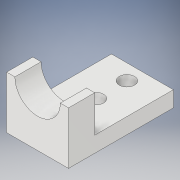
# Autodesk Inventor part: IndicatorLightMount
Saved by Autodesk Inventor 2018 (Build 220112000, 112)
## iProperties
Created: 2019-04-15
Part Number: IndicatorLightMount
Material: Generic
Document SubType Name: Modeling
Designer: anirudh
Density: 1 g/cm^3
Appearance: White
Mass: 2.43229 g
Surface Area: 18.7803 cm^2
Volume: 2.43229 cm^3
Author: anirudh
Autodesk Inventor part; units mm, degrees
ref_plane "YZ Plane" through (0, 0, 0) normal (1, 0, 0) x (0, 1, 0)
ref_plane "XZ Plane" through (0, 0, 0) normal (0, 1, 0) x (-1, 0, 0)
ref_plane "XY Plane" through (0, 0, 0) normal (0, 0, 1) x (1, 0, 0)
sketch "Sketch1" plane through (0, 0, 0) normal (0, 1, 0) x (-1, 0, 0)
  line L0 (0, 0) -> (15, 0)
  line L1 (15, 0) -> (15, 25.4)
  line L2 (15, 25.4) -> (0, 25.4)
  line L3 (0, 25.4) -> (0, 0)
  dimension "d0" = 15
  dimension "d1" = 25.4
  constraints: 8 end point, 2 parallel, 1 horizontal, 1 perpendicular
  measures "d0" distance of L2.end L1.end
  measures "d1" distance of L1.end L0.end
extrude "Extrusion1" add sketch "Sketch1" along normal blind 6.35
sketch "Sketch2" plane through (0, 6.35, 0) normal (0, 1, 0) x (1, 0, 0)
  line L0 (-15, 0) -> (-15, -25.4) projected
  line L1 (0, -25.4) -> (0, 0) projected
  line L2 (-15, -25.4) -> (0, -25.4)
  line L3 (0, -25.4) -> (0, -19.05)
  line L4 (0, -19.05) -> (-15, -19.05)
  line L5 (-15, -19.05) -> (-15, -25.4)
  dimension "d4" = 6.35
  constraints: 8 end point, 2 parallel, 1 horizontal, 1 perpendicular, 1 point on line
  measures "d4" distance of L3.end L2.end
extrude "Extrusion2" add sketch "Sketch2" along normal blind 12.7
sketch "Sketch3" plane through (-15, 0, 25.4) normal (0, 0, 1) x (1, 0, 0)
  line L0 (0, 0) -> (0, 19.05) projected
  line L1 (15, 0) -> (15, 19.05) projected
  circle A0 centre (7.5, 12.7) radius 5.5
  dimension "d8" = 11
  constraints: 1 centre point
  measures "d8" diameter of A0
extrude "Extrusion3" cut sketch "Sketch3" against normal blind 12.7
sketch "Sketch4" plane through (0, 19.05, 0) normal (0, 1, 0) x (1, 0, 0)
  line L0 (0, -19.05) -> (-15, -19.05) projected
  line L1 (-15, -25.4) -> (0, -25.4)
  line L2 (0, -25.4) -> (0, -19.05)
  line L3 (0, -19.05) -> (-15, -19.05)
  line L4 (-15, -19.05) -> (-15, -25.4)
  point P0 (0, 0)
  constraints: 8 end point, 2 parallel, 1 horizontal, 1 perpendicular
extrude "Extrusion4" add sketch "Sketch4" along normal blind 2.54
sketch "Sketch5" plane through (0, 6.35, 0) normal (0, 1, 0) x (1, 0, 0)
  line L0 (0, 0) -> (-15, 0) projected
  line L1 (-15, -19.05) -> (0, -19.05) projected
  line L2 (-15, 0) -> (0, 0)
  line L3 (0, 0) -> (0, -19.05)
  line L4 (0, -19.05) -> (-15, -19.05)
  line L5 (-15, -19.05) -> (-15, 0)
  constraints: 8 end point, 2 parallel, 1 horizontal, 1 perpendicular
extrude "Extrusion5" cut sketch "Sketch5" against normal blind 2.54
sketch "Sketch6" plane through (0, 3.81, 0) normal (0, 1, 0) x (1, 0, 0)
  circle A0 centre (-7.5, -11.25) radius 1.85
  circle A1 centre (-7.5, -3.75) radius 1.85
  point P0 (0, 0)
  point P1 (-15, 0)
  dimension "d18" = 3.7
  dimension "d19" = 3.7
  constraints: 2 centre point
  measures "d18" diameter of A0
  measures "d19" diameter of A1
extrude "Extrusion6" cut sketch "Sketch6" against normal blind 8.89
sketch "Sketch7" plane through (-15, 0, 25.4) normal (0, 0, 1) x (1, 0, 0)
  circle A0 centre (7.5, 12.7) radius 5.5 projected
  line L0 (2, 12.7) -> (2, 21.59)
  line L1 (15, 21.59) -> (0, 21.59) projected
  line L2 (2, 12.7) -> (13, 12.7)
  line L3 (13, 12.7) -> (13, 21.59)
  line L4 (2, 21.59) -> (13, 21.59)
  point P0 (15, 0)
  constraints: 8 end point, 2 perpendicular, 2 point on circle, 2 point on line, 1 collinear, 1 vertical
extrude "Extrusion7" cut sketch "Sketch7" against normal blind 25.4 contours L2 A0 | A0 L0 L1 L3 picked at (8.1501, 14.4142)
sketch "Sketch8" plane through (-15, 0, 25.4) normal (0, 0, 1) x (1, 0, 0)
  line L0 (0, 0) -> (0, 21.59) projected
  line L1 (0, 21.59) -> (15, 21.59)
  line L2 (15, 21.59) -> (15, 12.7)
  line L3 (15, 12.7) -> (0, 12.7)
  line L4 (0, 12.7) -> (0, 21.59)
  point P0 (15, 0)
  constraints: 8 end point, 2 parallel, 1 horizontal, 1 perpendicular
extrude "Extrusion8" cut sketch "Sketch8" against normal blind 25.4
body "Solid1"
